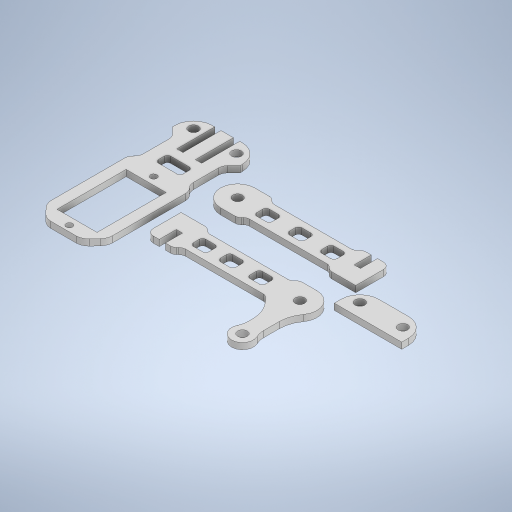
# Autodesk Inventor part: carbon_tail_parts
Saved by Autodesk Inventor 2024 (Build 280153000, 153)
## iProperties
Created: 2024-04-09
Part Number: carbon_tail_parts
Material: Generic
Document SubType Name: Modeling
Designer: nikop
Density: 1 g/cm^3
Appearance: Default
Author: nikop
Autodesk Inventor part; units mm, degrees
ref_plane "YZ Plane" through (0, 0, 0) normal (1, 0, 0) x (0, 1, 0)
ref_plane "XZ Plane" through (0, 0, 0) normal (0, 1, 0) x (-1, 0, 0)
ref_plane "XY Plane" through (0, 0, 0) normal (0, 0, 1) x (1, 0, 0)
sketch "Sketch1" plane through (0, 0, 0) normal (0, 1, 0) x (-1, 0, 0)
  arc A0 (-12.2568, 18.9699) -> (-12.877, 16.2877) centre (-6.877, 16.3133) ccw
  arc A1 (-12.2421, 18.9673) -> (-18.5053, 18.9673) centre (-15.3737, 20.5303) ccw
  arc A2 (-17.877, 16.2877) -> (-18.512, 18.9664) centre (-23.877, 16.2799) ccw
  arc A3 (-19.8048, 5.3677) -> (-17.877, 11.2702) centre (-27.877, 11.2702) ccw
  arc A4 (-19.8157, 5.3702) -> (-15.3802, -3.3819) centre (-15.3802, 2.1181) ccw
  line L0 (-15.3802, -3.3819) -> (-10.7086, -3.3819)
  arc A5 (-10.7086, -3.3819) -> (-9.2944, -2.7962) centre (-10.7086, -1.3819) ccw
  line L1 (-9.2944, -2.7962) -> (-8.966, -2.4677)
  arc A6 (-7.5518, -1.8819) -> (-8.966, -2.4677) centre (-7.5518, -3.8819) ccw
  arc A7 (18.82, -2.4228) -> (17.4058, -1.837) centre (17.4058, -3.837) ccw
  line L2 (18.82, -2.4228) -> (19.1485, -2.7512)
  arc A8 (19.1485, -2.7512) -> (20.5627, -3.337) centre (20.5627, -1.337) ccw
  line L3 (20.5627, -3.337) -> (26.2343, -3.337)
  line L4 (24.2343, 2.163) -> (22.2343, 2.163)
  arc A9 (20.5627, 7.663) -> (19.1485, 7.0772) centre (20.5627, 5.663) ccw
  line L5 (19.1485, 7.0772) -> (18.82, 6.7488)
  arc A10 (17.4058, 6.163) -> (18.82, 6.7488) centre (17.4058, 8.163) ccw
  arc A11 (-8.966, 6.7038) -> (-7.5518, 6.1181) centre (-7.5518, 8.1181) ccw
  line L6 (-8.966, 6.7038) -> (-9.9513, 7.6891)
  arc A12 (-12.877, 14.7602) -> (-9.9179, 7.7017) centre (-2.8771, 14.8028) ccw
  arc A13 (16.7982, -21.072) -> (15.384, -20.4862) centre (15.384, -22.4862) ccw
  line L7 (16.7982, -21.072) -> (17.1266, -21.4005)
  arc A14 (17.1266, -21.4005) -> (18.5409, -21.9862) centre (18.5409, -19.9862) ccw
  line L8 (18.5409, -21.9862) -> (23.2124, -21.9862)
  arc A15 (23.2124, -21.9862) -> (28.7124, -16.4862) centre (23.2124, -16.4862) ccw
  arc A16 (28.7124, -16.4862) -> (23.2124, -10.9862) centre (23.2124, -16.4862) ccw
  line L9 (23.2124, -10.9862) -> (18.5409, -10.9862)
  arc A17 (18.5409, -10.9862) -> (17.1266, -11.572) centre (18.5409, -12.9862) ccw
  line L10 (17.1266, -11.572) -> (16.7982, -11.9005)
  arc A18 (15.384, -12.4862) -> (16.7982, -11.9005) centre (15.384, -10.4862) ccw
  arc A19 (-10.7404, -11.9586) -> (-9.6511, -12.5178) centre (-9.3262, -10.5444) ccw
  line L11 (-10.7404, -11.9586) -> (-11.0688, -11.6302)
  arc A20 (-11.0688, -11.6302) -> (-12.483, -11.0444) centre (-12.483, -13.0444) ccw
  line L12 (-12.483, -11.0444) -> (-18.1546, -11.0444)
  line L13 (-16.1546, -16.5444) -> (-14.1546, -16.5444)
  arc A21 (-12.483, -22.0444) -> (-11.0688, -21.4586) centre (-12.483, -20.0444) ccw
  line L14 (-11.0688, -21.4586) -> (-10.7404, -21.1302)
  arc A22 (-9.6332, -20.5681) -> (-10.7404, -21.1302) centre (-9.3262, -22.5444) ccw
  line L15 (4.1873, 2.0817) -> (4.1873, 3.0817)
  line L16 (4.1873, 2.0817) -> (4.1873, 1.0817)
  line L17 (17.8203, 2.163) -> (17.8203, 3.163)
  line L18 (17.8203, 2.163) -> (17.8203, 1.163)
  line L19 (13.8203, 0.163) -> (16.8203, 0.163)
  line L20 (28.2343, 2.163) -> (28.2343, 5.663)
  line L21 (28.2343, 2.163) -> (28.2343, -1.337)
  arc A23 (28.2284, 5.663) -> (26.2284, 7.663) centre (26.2284, 5.663) ccw
  arc A24 (17.8203, 3.163) -> (16.8203, 4.163) centre (16.8203, 3.163) ccw
  arc A25 (16.8203, 0.163) -> (17.8203, 1.163) centre (16.8203, 1.163) ccw
  arc A26 (5.1873, 4.0817) -> (4.1873, 3.0817) centre (5.1873, 3.0817) ccw
  arc A27 (4.1873, 1.0817) -> (5.1873, 0.0817) centre (5.1873, 1.0817) ccw
  line L22 (16.8203, 4.163) -> (13.8203, 4.163)
  line L23 (12.8203, 1.163) -> (12.8203, 3.163)
  line L24 (9.1873, 1.0817) -> (9.1873, 3.0817)
  line L25 (8.1873, 4.0817) -> (5.1873, 4.0817)
  line L26 (8.1873, 0.0817) -> (5.1873, 0.0817)
  arc A28 (13.8203, 4.163) -> (12.8203, 3.163) centre (13.8203, 3.163) ccw
  arc A29 (12.8203, 1.163) -> (13.8203, 0.163) centre (13.8203, 1.163) ccw
  arc A30 (9.1873, 3.0817) -> (8.1873, 4.0817) centre (8.1873, 3.0817) ccw
  arc A31 (8.1873, 0.0817) -> (9.1873, 1.0817) centre (8.1873, 1.0817) ccw
  line L27 (-20.1546, -16.5444) -> (-20.1546, -20.0444)
  line L28 (-20.1546, -16.5444) -> (-20.1546, -13.0444)
  arc A32 (-20.1546, -20.0444) -> (-18.1546, -22.0444) centre (-18.1546, -20.0444) ccw
  line L29 (16.0169, -16.4235) -> (16.0169, -17.4235)
  line L30 (16.0169, -16.4235) -> (16.0169, -15.4235)
  line L31 (-9.6805, -16.5444) -> (-9.6805, -17.5444)
  line L32 (-9.6805, -16.5444) -> (-9.6805, -15.5444)
  line L33 (-5.6805, -14.5444) -> (-8.6805, -14.5444)
  arc A33 (-9.6805, -17.5444) -> (-8.6805, -18.5444) centre (-8.6805, -17.5444) ccw
  arc A34 (-8.6805, -14.5444) -> (-9.6805, -15.5444) centre (-8.6805, -15.5444) ccw
  arc A35 (15.0169, -18.4235) -> (16.0169, -17.4235) centre (15.0169, -17.4235) ccw
  arc A36 (16.0169, -15.4235) -> (15.0169, -14.4235) centre (15.0169, -15.4235) ccw
  line L34 (-8.6805, -18.5444) -> (-5.6805, -18.5444)
  line L35 (-4.6805, -15.5444) -> (-4.6805, -17.5444)
  line L36 (11.0169, -15.4235) -> (11.0169, -17.4235)
  line L37 (12.0169, -18.4235) -> (15.0169, -18.4235)
  line L38 (12.0169, -14.4235) -> (15.0169, -14.4235)
  arc A37 (-5.6805, -18.5444) -> (-4.6805, -17.5444) centre (-5.6805, -17.5444) ccw
  arc A38 (-4.6805, -15.5444) -> (-5.6805, -14.5444) centre (-5.6805, -15.5444) ccw
  arc A39 (11.0169, -17.4235) -> (12.0169, -18.4235) centre (12.0169, -17.4235) ccw
  arc A40 (12.0169, -14.4235) -> (11.0169, -15.4235) centre (12.0169, -15.4235) ccw
  line L39 (20.5627, 7.663) -> (21.7343, 7.663)
  line L40 (24.7312, 7.663) -> (26.2284, 7.663)
  circle A41 centre (-15.3802, 2.1181) radius 1.55
  circle A42 centre (-15.3737, 20.5303) radius 1.55
  circle A43 centre (23.2124, -16.4862) radius 1.55
  line L41 (-18.1546, -22.0444) -> (-16.6546, -22.0444)
  line L42 (-13.6546, -22.0444) -> (-12.483, -22.0444)
  line L43 (-17.877, 16.2877) -> (-17.877, 11.2702)
  line L44 (-7.5518, 6.1181) -> (17.4482, 6.1181)
  line L45 (-7.5518, -1.8819) -> (17.4482, -1.8819)
  line L46 (-0.2319, 1.01) -> (-0.2319, 3.01)
  line L47 (-1.2319, 0.01) -> (-4.2319, 0.01)
  line L48 (-1.2319, 4.01) -> (-4.2319, 4.01)
  arc A44 (-0.2319, 3.01) -> (-1.2319, 4.01) centre (-1.2319, 3.01) ccw
  arc A45 (-1.2319, 0.01) -> (-0.2319, 1.01) centre (-1.2319, 1.01) ccw
  arc A46 (-4.2319, 4.01) -> (-5.2319, 3.01) centre (-4.2319, 3.01) ccw
  line L49 (-5.2319, 2.01) -> (-5.2319, 3.01)
  line L50 (-5.2319, 2.01) -> (-5.2319, 1.01)
  arc A47 (-5.2319, 1.01) -> (-4.2319, 0.01) centre (-4.2319, 1.01) ccw
  line L51 (15.384, -12.4862) -> (-9.616, -12.4862)
  line L52 (15.384, -20.4862) -> (-9.616, -20.4862)
  line L53 (0.6284, -16.462) -> (0.6284, -17.462)
  line L54 (1.6284, -18.462) -> (4.6284, -18.462)
  line L55 (0.6284, -16.462) -> (0.6284, -15.462)
  arc A48 (1.6284, -14.462) -> (0.6284, -15.462) centre (1.6284, -15.462) ccw
  arc A49 (0.6284, -17.462) -> (1.6284, -18.462) centre (1.6284, -17.462) ccw
  line L56 (5.6284, -15.462) -> (5.6284, -17.462)
  arc A50 (5.6284, -15.462) -> (4.6284, -14.462) centre (4.6284, -15.462) ccw
  arc A51 (4.6284, -18.462) -> (5.6284, -17.462) centre (4.6284, -17.462) ccw
  line L57 (4.6284, -14.462) -> (1.6284, -14.462)
  line L58 (26.2343, -3.337) -> (28.2343, -3.337)
  line L59 (28.2343, -3.337) -> (28.2343, -1.337)
  line L60 (-18.1546, -11.0444) -> (-20.1546, -11.0444)
  line L61 (-18.1546, -11.0444) -> (-16.1546, -11.0444) construction
  line L62 (-20.1546, -11.0444) -> (-20.1546, -13.0444)
  line L63 (21.8343, 7.663) -> (21.7343, 7.663)
  line L64 (24.6343, 7.663) -> (24.7312, 7.663)
  line L65 (-16.1546, -16.5444) -> (-15.7546, -16.5444) construction
  line L66 (-13.7546, -22.0444) -> (-13.6546, -22.0444)
  line L67 (-16.5546, -22.0444) -> (-16.6546, -22.0444)
  line L68 (22.2343, 2.163) -> (22.2343, 7.663)
  line L69 (22.2343, 7.663) -> (21.8343, 7.663)
  line L70 (24.2343, 2.163) -> (24.2343, 7.663)
  line L71 (24.2343, 7.663) -> (24.6343, 7.663)
  line L72 (-16.1546, -16.5444) -> (-16.1546, -22.0444)
  line L73 (-16.1546, -22.0444) -> (-16.5546, -22.0444)
  line L74 (-14.1546, -16.5444) -> (-14.1546, -22.0444)
  line L75 (-14.1546, -22.0444) -> (-13.7546, -22.0444)
  line L76 (31.7665, -25.818) -> (31.7665, -26.53)
  arc A52 (31.7665, -26.53) -> (37.7665, -32.53) centre (37.7665, -26.53) ccw
  line L77 (44.5915, -20.318) -> (46.5915, -20.318)
  arc A53 (47.4165, -32.53) -> (53.4165, -26.53) centre (47.4165, -26.53) ccw
  line L78 (53.4165, -26.53) -> (53.4165, -25.818)
  line L79 (48.0165, 15.72) -> (42.5915, 15.72)
  line L80 (42.5915, 15.72) -> (37.1665, 15.72)
  line L81 (31.7665, -25.818) -> (33.7128, -23.8717)
  line L82 (32.7665, 14.1472) -> (32.7665, -9.3134)
  line L83 (33.6452, -11.4347) -> (33.7128, -11.5023)
  line L84 (34.5915, -20.318) -> (34.5915, -21.7504)
  line L85 (34.5915, -20.318) -> (34.5915, -13.6237)
  line L86 (42.5915, 20.02) -> (38.5087, 20.02)
  line L87 (35.5799, 18.7444) -> (33.8378, 16.8716)
  arc A54 (38.5087, 20.02) -> (35.5799, 18.7444) centre (38.5087, 16.02) ccw
  arc A55 (33.8378, 16.8716) -> (32.7665, 14.1472) centre (36.7665, 14.1472) ccw
  arc A56 (33.7128, -23.8717) -> (34.5915, -21.7504) centre (31.5915, -21.7504) ccw
  arc A57 (34.5915, -13.6237) -> (33.7128, -11.5023) centre (31.5915, -13.6237) ccw
  arc A58 (32.7665, -9.3134) -> (33.6452, -11.4347) centre (35.7665, -9.3134) ccw
  line L88 (53.4165, -25.818) -> (51.4702, -23.8717)
  line L89 (52.4165, 14.1472) -> (52.4165, -9.3134)
  line L90 (51.5378, -11.4347) -> (51.4702, -11.5023)
  line L91 (50.5915, -20.318) -> (50.5915, -21.7504)
  line L92 (50.5915, -20.318) -> (50.5915, -13.6237)
  line L93 (42.5915, 20.02) -> (46.6744, 20.02)
  line L94 (49.6031, 18.7444) -> (51.3453, 16.8716)
  arc A59 (49.6031, 18.7444) -> (46.6744, 20.02) centre (46.6744, 16.02) ccw
  arc A60 (52.4165, 14.1472) -> (51.3453, 16.8716) centre (48.4165, 14.1472) ccw
  arc A61 (50.5915, -21.7504) -> (51.4702, -23.8717) centre (53.5915, -21.7504) ccw
  arc A62 (51.4702, -11.5023) -> (50.5915, -13.6237) centre (53.5915, -13.6237) ccw
  arc A63 (51.5378, -11.4347) -> (52.4165, -9.3134) centre (49.4165, -9.3134) ccw
  line L95 (38.5915, -16.318) -> (38.5915, -14.38)
  line L96 (39.5915, -13.38) -> (45.5915, -13.38)
  line L97 (39.5915, -17.318) -> (45.5915, -17.318)
  line L98 (46.5915, -16.318) -> (46.5915, -14.38)
  arc A64 (38.5915, -16.318) -> (39.5915, -17.318) centre (39.5915, -16.318) ccw
  arc A65 (39.5915, -13.38) -> (38.5915, -14.38) centre (39.5915, -14.38) ccw
  arc A66 (46.5915, -14.38) -> (45.5915, -13.38) centre (45.5915, -14.38) ccw
  arc A67 (45.5915, -17.318) -> (46.5915, -16.318) centre (45.5915, -16.318) ccw
  line L99 (37.7665, -32.53) -> (38.0915, -32.53)
  line L100 (37.1665, 15.72) -> (36.1665, 15.72)
  line L101 (48.0165, 15.72) -> (49.0165, 15.72)
  line L102 (36.1665, 15.72) -> (36.1665, -6.48)
  line L103 (49.0165, 15.72) -> (49.0165, -6.48)
  line L104 (36.1665, -6.48) -> (49.0165, -6.48)
  line L105 (44.5915, -20.318) -> (45.0915, -20.318) construction
  line L106 (46.5915, -20.318) -> (47.0915, -20.318) construction
  line L107 (47.4165, -32.53) -> (47.0915, -32.53)
  line L108 (41.0915, -32.53) -> (44.0915, -32.53)
  circle A68 centre (49.4915, -28.618) radius 1.55
  circle A69 centre (35.6915, -28.618) radius 1.55
  circle A70 centre (42.5915, -8.93) radius 1.05
  circle A71 centre (42.5915, 18.17) radius 1.05
  line L109 (38.5915, -20.318) -> (38.5915, -32.53)
  line L110 (38.5915, -32.53) -> (38.0915, -32.53)
  line L111 (40.5915, -20.318) -> (40.5915, -32.53)
  line L112 (40.5915, -32.53) -> (41.0915, -32.53)
  line L113 (38.5915, -20.318) -> (40.5915, -20.318)
  line L114 (44.5915, -20.318) -> (44.5915, -32.53)
  line L115 (44.5915, -32.53) -> (44.0915, -32.53)
  line L116 (46.5915, -20.318) -> (46.5915, -32.53)
  line L117 (46.5915, -32.53) -> (47.0915, -32.53)
  line L118 (-21.6171, -4.9214) -> (-21.6171, -4.2095)
  line L119 (-43.2671, -4.2095) -> (-43.2671, -4.9214)
  arc A72 (-43.2671, -4.9214) -> (-37.2671, -10.9214) centre (-37.2671, -4.9214) ccw
  line L120 (-37.2671, -10.9214) -> (-27.6171, -10.9214)
  arc A73 (-27.6171, -10.9214) -> (-21.6171, -4.9214) centre (-27.6171, -4.9214) ccw
  circle A74 centre (-39.3421, -7.0095) radius 1.55
  circle A75 centre (-25.5421, -7.0095) radius 1.55
  line L121 (-43.2671, -4.2095) -> (-43.2671, -2.7095)
  line L122 (-21.6171, -4.2095) -> (-21.6171, -2.7095)
  line L123 (-43.2671, -2.7095) -> (-21.6171, -2.7095)
  line L124 (17.4058, 6.163) -> (17.4482, 6.1181)
  line L125 (28.2284, 5.663) -> (28.2343, 5.663)
  line L126 (17.4058, -1.837) -> (17.4482, -1.8819)
  line L127 (-9.6332, -20.5681) -> (-9.616, -20.4862)
  line L128 (-9.6511, -12.5178) -> (-9.616, -12.4862)
  line L129 (-9.9513, 7.6891) -> (-9.9179, 7.7017)
  line L130 (-19.8157, 5.3702) -> (-19.8048, 5.3677)
  line L131 (-12.877, 14.7602) -> (-12.877, 16.2877)
  line L132 (-12.2568, 18.9699) -> (-12.2421, 18.9673)
  line L133 (-18.5053, 18.9673) -> (-18.512, 18.9664)
  point P0 (0, 0)
  point P1 (52.4165, 14.1472)
  point P2 (49.6031, 18.7444)
  point P3 (46.6744, 20.02)
  point P4 (35.5799, 18.7444)
  point P5 (53.4165, -26.53)
  point P6 (51.4702, -23.8717)
  point P7 (45.5915, -13.38)
  point P8 (46.5915, -14.38)
  point P9 (39.5915, -17.318)
  point P10 (16.7982, -21.072)
  point P11 (23.2124, -21.9862)
  point P12 (28.7124, -16.4862)
  point P13 (23.2124, -10.9862)
  point P14 (-12.483, -11.0444)
  point P15 (-11.0688, -21.4586)
  point P16 (0.6284, -15.462)
  point P17 (4.6284, -14.462)
  point P18 (5.6284, -15.462)
  point P19 (0.6284, -17.462)
  point P20 (-37.2671, -10.9214)
  point P21 (-15.3802, -3.3819)
  point P22 (-9.2944, -2.7962)
  point P23 (18.82, -2.4228)
  point P24 (20.5627, -3.337)
  point P25 (19.1485, 7.0772)
  point P26 (-8.966, 6.7038)
  point P27 (-4.2319, 4.01)
  point P28 (-0.2319, 1.01)
  point P29 (-4.2319, 0.01)
  point P30 (-5.2319, 1.01)
  point P31 (4.1873, 3.0817)
  point P32 (5.1873, 4.0817)
  point P33 (8.1873, 4.0817)
  point P34 (8.1873, 0.0817)
  point P35 (5.1873, 0.0817)
  point P36 (4.1873, 1.0817)
  point P37 (12.8203, 1.163)
  point P38 (16.8203, 4.163)
  point P39 (17.8203, 1.163)
  point P40 (16.8203, 0.163)
  dimension "d0" = 3.1
  dimension "d1" = 3.1
  dimension "d2" = 3.1
  dimension "d3" = 25
  dimension "d4" = 25
  dimension "d5" = 25
  dimension "d6" = 2
  dimension "d7" = 180
  dimension "d8" = 1
  dimension "d9" = 1
  dimension "d10" = 22.2
  dimension "d11" = 22.2
  dimension "d12" = 3.1
  dimension "d13" = 3.1
  dimension "d14" = 2.1
  dimension "d15" = 2.1
  dimension "d16" = 3.1
  dimension "d17" = 3.1
  dimension "d18" = 1.5
  dimension "d19" = 1.5
  constraints: 268 end point, 134 point on circle, 76 centre point, 21 horizontal, 13 perpendicular, 10 vertical, 4 collinear, 3 point on line, 1 parallel, 1 tangent
  measures "d0" diameter of A41
  measures "d1" diameter of A42
  measures "d2" diameter of A43
  measures "d3" distance of L44.start L44.end
  measures "d4" distance of L45.start L45.end
  measures "d5" distance of L52.start L52.end
  measures "d6" distance of L12.end L60.end
  measures "d7" angle of L60 L61
  measures "d8" distance of L80.end L100.end
  measures "d9" distance of L101.start L101.end
  measures "d10" distance of L100.end L104.start
  measures "d11" distance of L101.end L103.end
  measures "d12" diameter of A68
  measures "d13" diameter of A69
  measures "d14" diameter of A70
  measures "d15" diameter of A71
  measures "d16" diameter of A74
  measures "d17" diameter of A75
  measures "d18" distance of L119.start L121.end
  measures "d19" distance of L122.start L122.end
extrude "Extrusion1" add sketch "Sketch1" along normal blind 2
body "Solid1"
